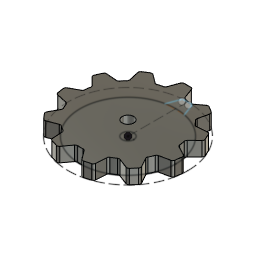
Gear_Template v0 (Autodesk Fusion 360 design; units mm, degrees)
Autodesk Fusion 360 part; units mm, degrees
sketch "Sketch1" plane through (0, 0, 0) normal (0, 0, 1) x (1, 0, 0)
  circle A0 centre (0, 0) radius 1.2
  circle A1 centre (0, 0) radius 10
  circle A2 centre (0, 0) radius 12.5 construction
  line L0 (0, 0) -> (0, 12.5) construction
  line L1 (-1.1518, 12.1283) -> (-2, 9.798)
  line L2 (1.1518, 12.1283) -> (2, 9.798)
  line L3 (-2, 9.798) -> (2, 9.798) construction
  line L4 (-0.682, 12.4573) -> (0.682, 12.4573)
  arc A3 (-0.682, 12.4573) -> (-1.1518, 12.1283) centre (-0.682, 11.9573) ccw
  arc A4 (1.1518, 12.1283) -> (0.682, 12.4573) centre (0.682, 11.9573) ccw
  dimension "d4" = 2.4
  dimension "d5" = 20
  dimension "d6" = 25
  dimension "d12" = 70
  dimension "d14" = 4
  dimension "d24" = 0.5
  constraint coincident A0.centre A1.centre
  constraint concentric A0 A2
  constraint coincident A2 L0.end
  constraint vertical L0
  constraint coincident A1 L1.end
  constraint coincident A1 L2.end
  constraint symmetric L0 L1 L2
  constraint tangent L4 A3
  constraint tangent L1 A3
  constraint symmetric L0 L4.start L4.end
  constraint symmetric L0 L1.start L2.start
  constraint symmetric L0 A3 A4
  measures "d4" diameter of A0
  measures "d5" diameter of A1
  measures "d6" diameter of A2
  measures "d12" angle of L1 L3
  measures "d14" distance of L1.end L2.end
  measures "d24" radius of A3
extrude "Extrude1" add sketch "Sketch1" along normal blind 3 contours A1
extrude "Extrude2" add sketch "Sketch1" along normal blind 3 contours A1 L1 L2 L4 A3 A4
fillet "Fillet1" radius 0.5 2 edges at (-2, 9.798, 1.5) (2, 9.798, 1.5)
pattern_circular "C-Pattern2" count 11 over 360 about axis through (0, 0, 3) along (0, 0, 1) of "Extrude2", "Fillet1"
equation "Rod_Diameter = 2.4 mm"
equation "Gear_Diameter = 20 mm"
equation "Teeth_Diameter = 25 mm"
equation "d4 = Rod_Diameter"
equation "d5 = Gear_Diameter"
equation "d6 = Teeth_Diameter"
equation "Tooth_Angle = 70 deg"
equation "d12 = Tooth_Angle"
equation "Tooth_Base = 4 mm"
equation "d14 = Tooth_Base"
equation "d16 = Gear_Thickness"
equation "d18 = Gear_Thickness"
equation "Tooth_Number = 11"
equation "Gear_Thickness = 3 mm"
equation "d24 = Fillet_Radius"
equation "Fillet_Radius = 0.5 mm"
equation "d28 = Fillet_Radius"
equation "d29 = Tooth_Number"
